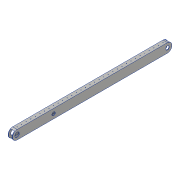
# Autodesk Inventor part: Support Pivs 25 middle
Saved by Autodesk Inventor 2018 (Build 220112000, 112)
## iProperties
Created: 2018-01-08
Part Number: Support Pivs 25 middle
Material: Aluminum 6061
Document SubType Name: Modeling
Designer: dsayers
Density: 2.7 g/cm^3
Appearance: Aluminum - Flat
Mass: 832.143 g
Surface Area: 2463.38 cm^2
Volume: 308.201 cm^3
Author: dsayers
Autodesk Inventor part; units mm, degrees
ref_plane "YZ Plane" through (0, 0, 0) normal (1, 0, 0) x (0, 1, 0)
ref_plane "XZ Plane" through (0, 0, 0) normal (0, 1, 0) x (-1, 0, 0)
ref_plane "XY Plane" through (0, 0, 0) normal (0, 0, 1) x (1, 0, 0)
sketch "Sketch1" plane through (0, 0, 0) normal (0, 0, 1) x (1, 0, 0)
  line L0 (0, 0) -> (25.4, 0)
  line L1 (25.4, 0) -> (25.4, 50.8)
  line L2 (25.4, 50.8) -> (0, 50.8)
  line L3 (0, 50.8) -> (0, 0)
  dimension "d0" = 25.4
  dimension "d1" = 50.8
  constraints: 8 end point, 2 parallel, 1 horizontal, 1 perpendicular
  measures "d0" distance of L1.end L2.end
  measures "d1" distance of L0.end L1.end
extrude "Extrusion1" add sketch "Sketch1" along normal blind 889
shell "Shell1" thickness 2.54 removed faces 2 at (8.4667, 33.8667, 889) at (8.4667, 33.8667, 0)
sketch "Sketch2" plane through (0, 50.8, 0) normal (0, 1, 0) x (1, 0, 0)
  line L0 (25.4, 0) -> (0, 0) projected
  line L1 (0, 0) -> (0, -889) projected
  point P0 (12.7, -12.7)
  point P1 (12.7, -38.1)
  point P2 (12.7, -63.5)
  point P3 (12.7, -88.9)
  point P4 (12.7, -114.3)
  point P5 (12.7, -139.7)
  point P6 (12.7, -165.1)
  point P7 (12.7, -190.5)
  point P8 (12.7, -215.9)
  point P9 (12.7, -241.3)
  point P10 (12.7, -266.7)
  point P11 (12.7, -292.1)
  point P12 (12.7, -317.5)
  point P13 (12.7, -342.9)
  point P14 (12.7, -368.3)
  point P15 (12.7, -393.7)
  point P16 (12.7, -419.1)
  point P17 (12.7, -444.5)
  point P18 (12.7, -469.9)
  point P19 (12.7, -495.3)
  point P20 (12.7, -520.7)
  point P21 (12.7, -546.1)
  point P22 (12.7, -571.5)
  point P23 (12.7, -596.9)
  point P24 (12.7, -622.3)
  point P25 (12.7, -647.7)
  point P26 (12.7, -673.1)
  point P27 (12.7, -698.5)
  point P28 (12.7, -723.9)
  point P29 (12.7, -749.3)
  point P30 (12.7, -774.7)
  point P31 (12.7, -800.1)
  point P32 (12.7, -825.5)
  point P33 (12.7, -850.9)
  point P34 (12.7, -876.3)
  point P35 (12.7, -901.7)
  point P36 (12.7, -927.1)
  dimension "d5" = 12.7
  dimension "d6" = 12.7
  dimension "d9" = 25.4
  constraints: 1 vertical, 36 other
  measures "d5" distance from line of L0 point (12.7, -12.7)
  measures "d6" distance from line of L1 point (12.7, -12.7)
  measures "d9" distance of point (12.7, -12.7) point (12.7, -38.1)
hole "Hole1" at (12.7, 50.8, 12.7) at (12.7, 50.8, 38.1) at (12.7, 50.8, 63.5) at (12.7, 50.8, 88.9) at (12.7, 50.8, 114.3) at (12.7, 50.8, 139.7) at (12.7, 50.8, 165.1) at (12.7, 50.8, 190.5) at (12.7, 50.8, 215.9) at (12.7, 50.8, 241.3) at (12.7, 50.8, 266.7) at (12.7, 50.8, 292.1) at (12.7, 50.8, 317.5) at (12.7, 50.8, 342.9) at (12.7, 50.8, 368.3) at (12.7, 50.8, 393.7) at (12.7, 50.8, 419.1) at (12.7, 50.8, 444.5) at (12.7, 50.8, 469.9) at (12.7, 50.8, 495.3) at (12.7, 50.8, 520.7) at (12.7, 50.8, 546.1) at (12.7, 50.8, 571.5) at (12.7, 50.8, 596.9) at (12.7, 50.8, 622.3) at (12.7, 50.8, 647.7) at (12.7, 50.8, 673.1) at (12.7, 50.8, 698.5) at (12.7, 50.8, 723.9) at (12.7, 50.8, 749.3) at (12.7, 50.8, 774.7) at (12.7, 50.8, 800.1) at (12.7, 50.8, 825.5) at (12.7, 50.8, 850.9) at (12.7, 50.8, 876.3) at (12.7, 50.8, 901.7) direction (0, -1, 0) diameter 2.54 depth 50.8 tip angle 118
sketch "Sketch6" plane through (25.4, 0, 0) normal (1, 0, 0) x (0, 0, -1)
  line L0 (0, 50.8) -> (-889, 50.8) projected
  line L1 (-889, 0) -> (-889, 50.8) projected
  line L2 (-869.0993, 34.925) -> (-858.1007, 34.925)
  line L3 (-858.1007, 34.925) -> (-852.6015, 25.4)
  line L4 (-852.6015, 25.4) -> (-858.1007, 15.875)
  line L5 (-858.1007, 15.875) -> (-869.0993, 15.875)
  line L6 (-869.0993, 15.875) -> (-874.5985, 25.4)
  line L7 (-874.5985, 25.4) -> (-869.0993, 34.925)
  point P0 (0, 0)
  point P1 (-863.6, 25.4)
  point P2 (-863.6, 25.4)
  dimension "d48" = 25.4
  dimension "d49" = 25.4
  dimension "d50" = 19.05
  constraints: 12 end point, 1 coincident, 1 parallel, 13 other
  measures "d48" distance from line of L0 point (-863.6, 25.4)
  measures "d49" distance from line of L1 point (-863.6, 25.4)
  measures "d50" distance between parallel lines of L5 L2
extrude "Extrusion2" cut sketch "Sketch6" against normal blind 25.4
sketch "Sketch7" plane through (25.4, 0, 0) normal (1, 0, 0) x (0, 0, -1)
  line L0 (-869.0993, 34.925) -> (-858.1007, 34.925) projected
  line L1 (-874.5985, 25.4) -> (-869.0993, 34.925) projected
  line L2 (-869.0993, 34.925) -> (-858.1007, 34.925) projected
  line L3 (-858.1007, 34.925) -> (-852.6015, 25.4) projected
  line L4 (-852.6015, 25.4) -> (-858.1007, 15.875) projected
  line L5 (-858.1007, 15.875) -> (-869.0993, 15.875) projected
  line L6 (-869.0993, 15.875) -> (-874.5985, 25.4) projected
  line L7 (0, 0) -> (0, 50.8) projected
  line L8 (0, 50.8) -> (-889, 50.8) projected
  line L9 (-889, 0) -> (-889, 50.8) projected
  line L10 (0, 0) -> (-889, 0) projected
  arc A0 (-863.6, 50.8) -> (-863.6, 0) centre (-863.6, 25.4) ccw
  line L11 (-863.6, 50.8) -> (-889, 50.8)
  line L12 (-598.17, 48.26) -> (-598.17, 50.8) projected
  line L13 (-889, 50.8) -> (-889, 25.4)
  line L14 (-889, 48.26) -> (-889, 2.54) projected
  line L15 (-889, 0) -> (-889, 25.4)
  line L16 (-889, 0) -> (-863.6, 0)
  line L17 (-889, 0) -> (-889, 50.8) projected
  line L18 (-863.6, 50.8) -> (-889, 50.8)
  line L19 (-889, 50.8) -> (-889, 25.4)
  line L20 (-889, 2.54) -> (-889, 48.26) projected
  line L21 (0, 0) -> (-889, 0) projected
  arc A1 (-863.6, 50.8) -> (-761.9714, 0) centre (-863.6, -76.2573) ccw
  dimension "d53" = 10.9985
  dimension "d54" = 10.9985
  constraints: 12 end point, 5 point on circle, 3 point on line, 2 centre point, 2 midpoint, 2 perpendicular, 2 tangent, 1 coincident, 1 collinear
  measures "d53" distance of L1.start point (-863.6, 25.4)
  measures "d54" distance of L3.end point (-863.6, 25.4)
extrude "Extrusion3" cut sketch "Sketch7" against normal blind 25.4 contours L10 L9 A0 | A1 A0 L9 | L9 L8 A1
sketch "Sketch8" plane through (25.4, 0, 0) normal (1, 0, 0) x (0, 0, -1)
  line L0 (-19.9007, 15.875) -> (-30.8993, 15.875)
  line L1 (-30.8993, 15.875) -> (-36.3985, 25.4)
  line L2 (-36.3985, 25.4) -> (-30.8993, 34.925)
  line L3 (-30.8993, 34.925) -> (-19.9007, 34.925)
  line L4 (-19.9007, 34.925) -> (-14.4015, 25.4)
  line L5 (-14.4015, 25.4) -> (-19.9007, 15.875)
  line L6 (0, 50.8) -> (-863.6, 50.8) projected
  line L7 (0, 0) -> (0, 50.8) projected
  point P0 (-25.4, 25.4)
  dimension "d57" = 25.4
  dimension "d58" = 19.05
  dimension "d59" = 25.4
  constraints: 12 end point, 1 parallel, 13 other
  measures "d57" distance from line of L6 point (-25.4, 25.4)
  measures "d58" distance between parallel lines of L0 L3
  measures "d59" distance from line of L7 point (-25.4, 25.4)
extrude "Extrusion4" cut sketch "Sketch8" against normal blind 25.4
fillet "Fillet1" radius 25.4 2 edges at (12.7, 50.8, 0) (12.7, 0, 0)
sketch "Sketch9" plane through (25.4, 25.4, 863.6) normal (1, 0, 0) x (0, 0, -1)
  line L0 (849.1985, 0) -> (843.6993, -9.525) projected
  line L1 (843.6993, -9.525) -> (832.7007, -9.525) projected
  line L2 (832.7007, -9.525) -> (827.2015, 0) projected
  line L3 (827.2015, 0) -> (832.7007, 9.525) projected
  line L4 (832.7007, 9.525) -> (843.6993, 9.525) projected
  line L5 (843.6993, 9.525) -> (849.1985, 0) projected
  arc A0 (838.2, -25.4) -> (838.2, 25.4) centre (838.2, 0) ccw projected
  line L6 (838.2, 25.4) -> (0, 25.4) projected
  arc A1 (0, 25.4) -> (0, -25.4) centre (0, 0) ccw projected
  line L7 (838.2, -25.4) -> (0, -25.4) projected
  line L8 (-10.9985, 0) -> (-5.4993, 9.525) projected
  line L9 (-5.4993, 9.525) -> (5.4993, 9.525) projected
  line L10 (5.4993, 9.525) -> (10.9985, 0) projected
  line L11 (10.9985, 0) -> (5.4993, -9.525) projected
  line L12 (5.4993, -9.525) -> (-5.4993, -9.525) projected
  line L13 (-5.4993, -9.525) -> (-10.9985, 0) projected
  circle A2 centre (0, 0) radius 12.7
  point P0 (863.6, -25.4)
  dimension "d63" = 25.4
  constraints: 1 centre point, 1 coincident
  measures "d63" diameter of A2
extrude "Extrusion5" cut sketch "Sketch9" against normal blind 25.4 contours A2
sketch "Sketch10" plane through (25.4, 25.4, 863.6) normal (1, 0, 0) x (0, 0, -1)
  circle A0 centre (0, 0) radius 12.7 projected
  point P0 (863.6, -25.4)
  point P1 (203.2, -0.6062)
  dimension "d66" = 203.2
  measures "d66" horizontal distance of A0.centre point (203.2, -0.606)
hole "Hole5" at (25.4, 24.7938, 660.4) direction (-1, 0, 0) diameter 19.05 depth 25.4 tip angle 118
body "Solid1"
